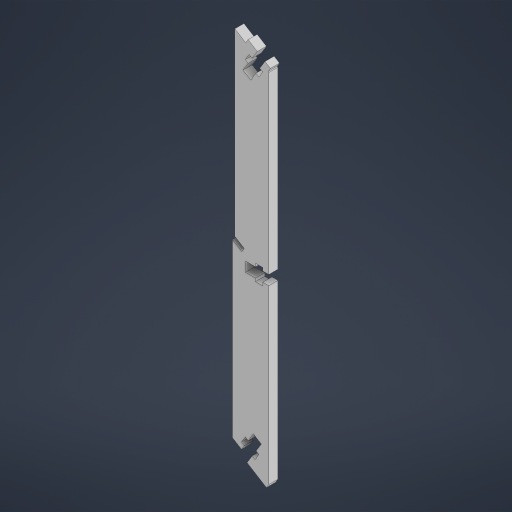
# Autodesk Inventor part: Inner Bracket
Saved by Autodesk Inventor 2023 (Build 270158000, 158)
## iProperties
Created: 2022-06-20
Part Number: Inner Bracket
Material: Generic
Document SubType Name: Modeling
Designer: FizzyApple12
Density: 1 g/cm^3
Appearance: Default
Author: FizzyApple12
Autodesk Inventor part; units mm, degrees
ref_plane "YZ Plane" through (0, 0, 0) normal (1, 0, 0) x (0, 1, 0)
ref_plane "XZ Plane" through (0, 0, 0) normal (0, 1, 0) x (-1, 0, 0)
ref_plane "XY Plane" through (0, 0, 0) normal (0, 0, 1) x (1, 0, 0)
ref_plane "Work Plane1" through (0, 0, 0) normal (0, 0, 1) x (1, 0, 0)
sketch "Sketch1" plane through (0, 0, 0) normal (0, 0, 1) x (1, 0, 0)
  line L0 (-13.9399, 12.3161) -> (-5.7696, 7.2832) projected
  line L1 (-15.6051, 9.6128) -> (-13.9399, 12.3161) projected
  line L2 (-7.4348, 4.5799) -> (-15.6051, 9.6128) projected
  line L3 (-5.7696, 7.2832) -> (-7.4348, 4.5799) construction
  line L4 (-5.7696, 7.2832) -> (-3.8046, 6.0727) construction
  line L5 (-5.4698, 3.3694) -> (-7.4348, 4.5799) construction
  line L6 (-3.8046, 6.0727) -> (1.6652, 2.7033) projected
  line L7 (-5.4698, 3.3694) -> (-3.8046, 6.0727) construction
  line L8 (0, 0) -> (-5.4698, 3.3694) projected
  line L9 (0, 0) -> (1.6652, 2.7033) projected
  line L10 (-1.1208, -252.5481) -> (-16.3579, -243.162) projected
  line L11 (-14.6927, -240.4587) -> (0.5444, -249.8448) projected
  line L12 (-16.3579, -243.162) -> (-14.6927, -240.4587) construction
  line L13 (-9.0019, -247.6933) -> (-20.2167, -240.7849) construction
  line L14 (-6.6483, -245.4141) -> (-18.5515, -238.0817) construction
  line L15 (0.5444, -249.8448) -> (0.5444, -249.8448) projected
  ellipse E0 centre (0.5444, -126.068) end of major axis (0.5444, -129.4462) minor radius 0 construction
  line L16 (0.5444, -2.2912) -> (0.5444, 0.8838) construction
  line L17 (0.5444, 0.8838) -> (0.5444, 0.8838) construction
  line L18 (0.5444, 0.8838) -> (0.5444, -253.0198) construction
  line L19 (0.5444, -253.0198) -> (0.5444, -253.0198) construction
  line L20 (0.5444, -253.0198) -> (0.5444, 0.8838) construction
  line L21 (0.5444, 0.8838) -> (0.5444, 0.8838) construction
  line L22 (0.5444, 0.8838) -> (0.5444, -2.2912) construction
  line L23 (0.5444, -2.2912) -> (0.5444, -2.2912) construction
  line L24 (-7.4904, 8.3432) -> (-9.1556, 5.6399)
  line L25 (-3.7491, 2.3094) -> (-2.0838, 5.0127)
  line L26 (0, 0) -> (0.5444, -0.3354)
  line L27 (0.5444, -0.3354) -> (0.5444, -253.0198)
  line L28 (-2.1619, -248.1777) -> (0.5444, -249.8448)
  line L29 (-12.9719, -241.5187) -> (-14.6371, -244.222)
  line L30 (-15.6051, 9.6128) -> (-23.1742, 14.2754)
  line L31 (-23.1742, 14.2754) -> (-23.1742, -111.4572)
  line L32 (-25.9909, -237.228) -> (-24.3256, -234.5248) construction
  line L33 (-21.0892, -112.7416) -> (-23.1742, -111.4572) construction
  line L34 (-23.1742, -111.4572) -> (0.5444, -126.068) construction
  line L35 (-23.1742, -111.4572) -> (-24.8395, -114.1605) construction
  line L36 (-22.7544, -115.4449) -> (-24.8395, -114.1605) construction
  line L37 (-24.8395, -114.1605) -> (0.5444, -129.797) construction
  line L38 (-24.8395, -114.1605) -> (-24.8395, -234.2082)
  line L39 (-24.3256, -234.5248) -> (-24.8395, -234.2082) construction
  line L40 (-24.8395, -234.2082) -> (-18.5515, -238.0817)
  line L41 (-12.9719, -241.5187) -> (-4.6458, -228.0024)
  line L42 (-18.5515, -238.0817) -> (-10.2253, -224.5653)
  line L43 (-10.2253, -224.5653) -> (-4.6458, -228.0024)
  line L44 (-14.2208, -243.5461) -> (-0.7045, -251.8723)
  line L45 (1.2489, 2.0275) -> (-2.5002, 4.3369)
  line L46 (-7.9067, 7.6673) -> (-14.3562, 11.6402)
  ellipse E1 centre (0.5444, -126.068) end of major axis (0.5444, -129.4462) minor radius 0 construction
  line L47 (0.5444, -122.6898) -> (3.3735, -122.6898) construction
  line L48 (0.5444, -129.4462) -> (3.3735, -129.4462) construction
  ellipse E2 centre (3.3735, -126.068) end of major axis (3.3735, -129.4462) minor radius 0 construction
  line L49 (-3.7491, 2.3094) -> (-12.0752, -11.2069)
  line L50 (-12.0752, -11.2069) -> (-17.4817, -7.8765)
  line L51 (-17.4817, -7.8765) -> (-9.1556, 5.6399)
  line L52 (-14.7785, -9.5417) -> (-4.7871, 6.6779) construction
  line L53 (-15.8457, -0.6803) -> (-6.3842, -6.5086)
  line L54 (-6.3842, -6.5086) -> (-3.7199, -2.1834)
  line L55 (-3.7199, -2.1834) -> (-13.1813, 3.6449)
  line L56 (-13.1813, 3.6449) -> (-15.8457, -0.6803)
  line L57 (-15.8457, -0.6803) -> (-3.7199, -2.1834) construction
  line L58 (-6.3842, -6.5086) -> (-13.1813, 3.6449) construction
  line L59 (-7.4356, -226.2838) -> (-17.4269, -242.5035) construction
  line L60 (-18.4941, -233.6421) -> (-9.0327, -239.4704)
  line L61 (-9.0327, -239.4704) -> (-6.3683, -235.1452)
  line L62 (-6.3683, -235.1452) -> (-15.8298, -229.3169)
  line L63 (-15.8298, -229.3169) -> (-18.4941, -233.6421)
  line L64 (-18.4941, -233.6421) -> (-6.3683, -235.1452) construction
  line L65 (-9.0327, -239.4704) -> (-15.8298, -229.3169) construction
  line L66 (0.5444, -249.8448) -> (-1.1208, -252.5481) projected
  line L67 (0.5444, -122.6898) -> (-15.6765, -122.6898)
  line L68 (-15.6765, -122.6898) -> (-15.6765, -129.4462)
  line L69 (-15.6765, -129.4462) -> (0.5444, -129.4462)
  line L70 (3.3735, -126.068) -> (-15.6765, -126.068) construction
  line L71 (-8.6915, -131.6242) -> (-8.6915, -120.5117)
  line L72 (-8.6915, -120.5117) -> (-3.6115, -120.5117)
  line L73 (-3.6115, -120.5117) -> (-3.6115, -131.6242)
  line L74 (-3.6115, -131.6242) -> (-8.6915, -131.6242)
  line L75 (-8.6915, -131.6242) -> (-3.6115, -120.5117) construction
  line L76 (-8.6915, -120.5117) -> (-3.6115, -131.6242) construction
  line L77 (-24.8395, -114.1605) -> (-10.9932, -122.6898)
  line L78 (-23.1742, -111.4572) -> (-8.4754, -120.5117)
  line L79 (-16.6864, -115.4537) -> (-18.3516, -118.157)
  line L80 (-16.9504, 14.1706) -> (-18.6156, 11.4673) construction
  line L81 (-18.6156, 11.4673) -> (-23.1742, 4.067)
  line L82 (-23.2443, -111.414) -> (-24.9095, -114.1173) projected
  point P0 (-6.4523, 3.9747)
  point P1 (-9.7828, -1.4319)
  point P2 (-12.4312, -234.3936)
  point P3 (-6.1515, -126.068)
  point P4 (-16.5532, -234.8378)
  point P5 (-13.8888, -230.5125)
  point P6 (-8.3093, -233.9495)
  point P7 (-10.9736, -238.2748)
  point P8 (0.5444, -129.4462)
  point P9 (-3.6115, -129.4462)
  point P10 (-8.6915, -129.4462)
  point P11 (-8.6915, -122.6898)
  point P12 (-3.6115, -122.6898)
  point P13 (-5.7473, -0.9345)
  point P14 (-8.4117, -5.2597)
  point P15 (-13.8182, -1.9293)
  point P16 (-11.1539, 2.396)
  dimension "d0" = 3.175
  dimension "d1" = 3.175
  dimension "d2" = 2.021
  dimension "d3" = 2.021
  dimension "d5" = 19.05
  dimension "d7" = 0.7937
  dimension "d8" = 0.7937
  dimension "d9" = 19.05
  dimension "d10" = 8.89
  dimension "d11" = 11.1125
  dimension "d12" = 5.08
  dimension "d13" = 11.1125
  dimension "d14" = 5.08
  dimension "d15" = 19.05
  dimension "d16" = 11.1125
  dimension "d17" = 5.08
  dimension "d18" = 7.62
  constraints: 114 end point, 25 point on line, 17 perpendicular, 14 midpoint, 13 collinear, 13 parallel, 2 horizontal, 7 other
  measures "d0" distance from line of point (-6.452, 3.975) L25
  measures "d1" distance from line of L24 point (-6.452, 3.975)
  measures "d2" distance between parallel lines of L7 L25
  measures "d3" distance between parallel lines of L12 L29
  measures "d5" distance between parallel lines of L13 L43
  measures "d7" distance between parallel lines of L10 L44
  measures "d8" distance between parallel lines of L0 L46
  measures "d9" distance between parallel lines of L4 L50
  measures "d10" distance from line of L30.end L1
  measures "d11" distance of L53.start L53.end
  measures "d12" distance of L54.end L53.end
  measures "d13" distance of L60.start L60.end
  measures "d14" distance of L61.end L60.end
  measures "d15" distance from line of L70.start L68
  measures "d16" distance of L71.start L71.end
  measures "d17" distance of L71.end L72.end
  measures "d18" distance between parallel lines of L35 L79
extrude "Extrusion1" add sketch "Sketch1" along normal blind 6.35 contours L0 L24 L46 L1 | L46 L24 L2 L1 | L2 L51 L55 L56 L53 L50 L49 L54 L8 L26 L27 L67 L73 L72 L78 L31 L81 L30 | L81 L31 L30 | L25 L45 L9 L8 | L78 L72 L71 L67 L77 L79 | L25 L6 L9 L45 | L77 L67 L68 L69 L71 L74 L73 L27 L11 L41 L60 L61 L62 L43 L42 L63 L40 L38 | L66 L44 L29 L11 | L66 L10 L29 L44
equation "\"d1\" = d0"
equation "\"d3\" = d2"
body "Solid1"
